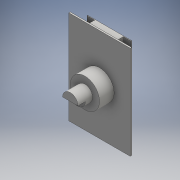
# Autodesk Inventor part: nasel_stand
Saved by Autodesk Inventor 2016 SP1 (Build 200210100, 210)
## iProperties
Created: 2017-01-27
Part Number: nasel_stand
Material: 一般
Document SubType Name: Modeling
Designer: p_admin
Density: 1 g/cm^3
Appearance: 既定
Author: p_admin
Autodesk Inventor part; units mm, degrees
ref_plane "YZ Plane" through (0, 0, 0) normal (1, 0, 0) x (0, 1, 0)
ref_plane "XZ Plane" through (0, 0, 0) normal (0, 1, 0) x (-1, 0, 0)
ref_plane "XY Plane" through (0, 0, 0) normal (0, 0, 1) x (1, 0, 0)
sketch "スケッチ1" plane through (0, 0, 0) normal (0, 0, 1) x (1, 0, 0)
  line L0 (-235, 10.2629) -> (65, 10.2629)
  line L1 (65, 10.2629) -> (65, 5.2629)
  line L2 (65, 5.2629) -> (-235, 5.2629)
  line L3 (-235, 5.2629) -> (-235, 10.2629)
  line L4 (-235, 10.2629) -> (65, 5.2629) construction
  line L5 (65, 10.2629) -> (-235, 5.2629) construction
  point P0 (0, 0)
  point P1 (-85, 7.7629)
  dimension "d0" = 300
  dimension "d1" = 5
  constraints: 12 end point, 2 midpoint, 2 parallel, 1 horizontal, 1 perpendicular
  measures "d0" distance of L1.end L2.end
  measures "d1" distance of L0.end L1.end
extrude "押し出し1" add sketch "スケッチ1" along normal blind 600
sketch "スケッチ2" plane through (-235, 5.2629, 0) normal (0, -1, 0) x (1, 0, 0)
  line L0 (50, 0) -> (250, 0)
  line L1 (250, 0) -> (250, 600)
  line L2 (250, 600) -> (50, 600)
  line L3 (50, 600) -> (50, 0)
  line L4 (300, 0) -> (0, 0) projected
  line L5 (0, 0) -> (0, 600) projected
  point P0 (235, 0)
  dimension "d4" = 200
  dimension "d5" = 600
  dimension "d6" = 0
  dimension "d7" = 50
  constraints: 8 end point, 2 parallel, 1 horizontal, 1 perpendicular
  measures "d4" distance of L2.end L1.end
  measures "d5" distance of L1.end L0.end
  measures "d6" distance between parallel lines of L4 L0
  measures "d7" distance between parallel lines of L5 L3
extrude "押し出し2" add sketch "スケッチ2" along normal blind 55
sketch "スケッチ3" plane through (-235, -49.7371, 0) normal (0, -1, 0) x (1, 0, 0)
  line L0 (-60, -20) -> (360, -20)
  line L1 (360, -20) -> (360, 620)
  line L2 (360, 620) -> (-60, 620)
  line L3 (-60, 620) -> (-60, -20)
  line L4 (0, 0) -> (300, 0) projected
  line L5 (0, 0) -> (0, 600) projected
  point P0 (235, 0)
  dimension "d10" = 420
  dimension "d11" = 640
  dimension "d12" = 20
  dimension "d13" = 60
  constraints: 8 end point, 2 parallel, 1 horizontal, 1 perpendicular
  measures "d10" distance of L2.end L1.end
  measures "d11" distance of L1.end L0.end
  measures "d12" distance between parallel lines of L4 L0
  measures "d13" distance between parallel lines of L5 L3
extrude "押し出し3" add sketch "スケッチ3" along normal blind 10
sketch "スケッチ4" plane through (-235, -49.7371, 0) normal (0, 1, 0) x (1, 0, 0)
  line L0 (-55, 2.2049) -> (355, 2.2049)
  line L1 (355, 2.2049) -> (355, 0)
  line L2 (355, 0) -> (-55, 0)
  line L3 (-55, 0) -> (-55, 2.2049)
  line L4 (-60, -620) -> (-60, 20) projected
  line L5 (-60, 20) -> (360, 20) projected
  line L6 (-55, -603) -> (355, -603)
  line L7 (355, -603) -> (355, -600)
  line L8 (355, -600) -> (-55, -600)
  line L9 (-55, -600) -> (-55, -603)
  line L10 (360, -620) -> (-60, -620) projected
  point P0 (235, 0)
  dimension "d16" = 410
  dimension "d17" = 5
  dimension "d18" = 20
  dimension "d19" = 410
  dimension "d20" = 3
  dimension "d21" = 20
  dimension "d22" = 5
  constraints: 16 end point, 4 parallel, 2 horizontal, 2 perpendicular
  measures "d16" distance of L2.end L1.end
  measures "d17" distance between parallel lines of L4 L3
  measures "d18" distance between parallel lines of L5 L2
  measures "d19" distance of L8.end L7.end
  measures "d20" distance of L7.end L6.end
  measures "d21" distance between parallel lines of L8 L10
  measures "d22" distance between parallel lines of L4 L9
extrude "押し出し4" cut sketch "スケッチ4" against normal blind 5
sketch "スケッチ5" plane through (15, 5.2629, 600) normal (1, 0, 0) x (0, 0, -1)
  line L0 (600, 0) -> (600, -55) projected
  line L1 (0, 0) -> (600, 0)
  line L2 (600, 0) -> (600, -55)
  line L3 (600, -55) -> (0, -55)
  line L4 (0, -55) -> (0, 0)
  point P0 (600, -5.2629)
  constraints: 8 end point, 2 parallel, 1 horizontal, 1 perpendicular
extrude "押し出し5" cut sketch "スケッチ5" against normal blind 2
sketch "スケッチ6" plane through (-185, 5.2629, 0) normal (-1, 0, 0) x (0, 0, 1)
  line L0 (0, 0) -> (600, 0) projected
  line L1 (-20, -55) -> (620, -55) projected
  line L2 (0, 0) -> (600, 0)
  line L3 (600, 0) -> (600, -55)
  line L4 (600, -55) -> (0, -55)
  line L5 (0, -55) -> (0, 0)
  point P0 (0, -5.2629)
  constraints: 8 end point, 2 parallel, 1 horizontal, 1 perpendicular, 1 point on line
extrude "押し出し6" cut sketch "スケッチ6" against normal blind 2
sketch "スケッチ7" plane through (-235, -59.7371, 0) normal (0, -1, 0) x (1, 0, 0)
  circle A0 centre (150, 300) radius 100
  line L0 (-60, 620) -> (-60, -20) projected
  line L1 (-60, -20) -> (360, -20) projected
  point P0 (235, 0)
  dimension "d29" = 200
  dimension "d30" = 210
  dimension "d31" = 320
  constraints: 1 centre point
  measures "d29" diameter of A0
  measures "d30" distance from line of L0 A0.centre
  measures "d31" distance from line of A0.centre L1
extrude "押し出し7" add sketch "スケッチ7" along normal blind 100
sketch "スケッチ8" plane through (-85, -159.7371, 300) normal (0, -1, 0) x (1, 0, 0)
  circle A0 centre (0, 0) radius 52.5
  point P0 (85, -300)
  dimension "d34" = 105
  constraints: 1 centre point
  measures "d34" diameter of A0
extrude "押し出し8" add sketch "スケッチ8" along normal blind 50
sketch "スケッチ9" plane through (-85, -209.7371, 300) normal (0, -1, 0) x (1, 0, 0)
  arc A0 (52.5, 0) -> (-52.5, 0) centre (0, 0) ccw
  line L0 (52.5, 0) -> (-52.5, 0)
  point P0 (85, -300)
  dimension "d37" = 105
  constraints: 2 end point, 2 point on circle, 1 centre point, 1 horizontal
  measures "d37" diameter of A0
extrude "押し出し9" add sketch "スケッチ9" along normal blind 50
